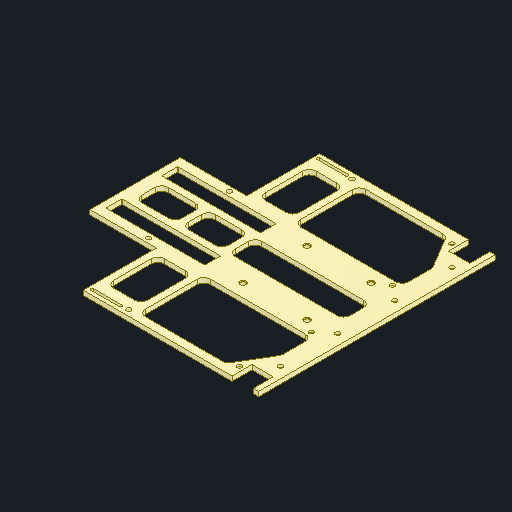
# Autodesk Inventor part: base
Saved by Autodesk Inventor 2023 (Build 270158000, 158)
## iProperties
Created: 2024-04-29
Part Number: base
Material: Nylon 6/6
Document SubType Name: Modeling
Designer: szymo
Density: 1.13 g/cm^3
Appearance: Nylon 6
Mass: 47.3407 g
Surface Area: 329.728 cm^2
Volume: 41.8944 cm^3
Author: szymo
Autodesk Inventor part; units mm, degrees
ref_plane "YZ Plane" through (0, 0, 0) normal (1, 0, 0) x (0, 1, 0)
ref_plane "XZ Plane" through (0, 0, 0) normal (0, 1, 0) x (-1, 0, 0)
ref_plane "XY Plane" through (0, 0, 0) normal (0, 0, 1) x (1, 0, 0)
sketch "Sketch1" plane through (0, 0, 0) normal (0, 1, 0) x (-1, 0, 0)
  line L0 (99, 89) -> (-99, 89)
  line L1 (-99, 89) -> (-99, -89)
  line L2 (-99, -89) -> (99, -89)
  line L3 (99, -89) -> (99, 89)
  line L4 (99, 89) -> (-99, -89) construction
  line L5 (-99, 89) -> (99, -89) construction
  line L6 (-99, 89) -> (-85, 89)
  line L7 (-85, 89) -> (-85, -89)
  line L8 (-85, -89) -> (-99, -89)
  line L9 (-99, -89) -> (-99, 89)
  line L10 (99, 89) -> (97, 89)
  line L11 (97, 89) -> (97, -89)
  line L12 (97, -89) -> (99, -89)
  line L13 (99, -89) -> (99, 89)
  line L14 (97, 33) -> (97, 35)
  line L15 (97, -33) -> (97, -35)
  line L16 (97, 32.8) -> (97, 35)
  line L17 (97, -32.8) -> (97, -35)
  line L18 (97, 89) -> (47, 89)
  line L19 (47, 89) -> (47, 34)
  line L20 (47, 34) -> (97, 34)
  line L21 (97, 34) -> (97, 89)
  line L22 (97, -89) -> (47, -89)
  line L23 (47, -89) -> (47, -34)
  line L24 (47, -34) -> (97, -34)
  line L25 (97, -34) -> (97, -89)
  line L26 (66.5, 33) -> (77.5, 33) projected
  line L27 (77.5, -33) -> (66.5, -33) projected
  line L28 (-81, 74) -> (-81, 89) projected
  line L29 (-81, 31) -> (-81, 55) projected
  line L30 (-81, -12) -> (-81, 12) projected
  line L31 (-81, -55) -> (-81, -31) projected
  line L32 (-81, -89) -> (-81, -74) projected
  arc A0 (-81, 74) -> (-79, 72) centre (-79, 74) ccw projected
  line L33 (-70, 72) -> (-79, 72) projected
  line L34 (-70, 57) -> (-70, 72) projected
  line L35 (-79, 57) -> (-70, 57) projected
  arc A1 (-79, 57) -> (-81, 55) centre (-79, 55) ccw projected
  arc A2 (-81, 31) -> (-79, 29) centre (-79, 31) ccw projected
  line L36 (-70, 29) -> (-79, 29) projected
  line L37 (-70, 14) -> (-70, 29) projected
  line L38 (-79, 14) -> (-70, 14) projected
  arc A3 (-79, 14) -> (-81, 12) centre (-79, 12) ccw projected
  arc A4 (-81, -12) -> (-79, -14) centre (-79, -12) ccw projected
  line L39 (-70, -14) -> (-79, -14) projected
  line L40 (-70, -29) -> (-70, -14) projected
  line L41 (-79, -29) -> (-70, -29) projected
  arc A5 (-79, -29) -> (-81, -31) centre (-79, -31) ccw projected
  arc A6 (-81, -55) -> (-79, -57) centre (-79, -55) ccw projected
  line L42 (-70, -57) -> (-79, -57) projected
  line L43 (-70, -72) -> (-70, -57) projected
  line L44 (-79, -72) -> (-70, -72) projected
  arc A7 (-79, -72) -> (-81, -74) centre (-79, -74) ccw projected
  circle A8 centre (-77, -64.5) radius 1.2295 projected
  circle A9 centre (-77, -21.5) radius 1.2295 projected
  circle A10 centre (-77, 21.5) radius 1.2295 projected
  circle A11 centre (-77, 64.5) radius 1.2295 projected
  line L45 (-65, 89) -> (-79, 89)
  line L46 (-79, 89) -> (-79, 75)
  line L47 (-79, 75) -> (-65, 75)
  line L48 (-65, 75) -> (-65, 89)
  line L49 (-65, 89) -> (-81, 89)
  line L50 (-81, 89) -> (-81, 74)
  line L51 (-81, 74) -> (-65, 74)
  line L52 (-65, 74) -> (-65, 89)
  line L53 (-99, 0) -> (97, 0)
  line L54 (0, 0) -> (-99, 0) construction
  line L55 (-65, -89) -> (-79, -89)
  line L56 (-79, -89) -> (-79, -75)
  line L57 (-79, -75) -> (-65, -75)
  line L58 (-65, -75) -> (-65, -89)
  line L59 (-65, -89) -> (-81, -89)
  line L60 (-81, -89) -> (-81, -74)
  line L61 (-81, -74) -> (-65, -74)
  line L62 (-65, -74) -> (-65, -89)
  point P0 (47, 89)
  point P1 (47, -89)
  point P2 (97, 34)
  point P3 (-81, -89)
  point P4 (-79, -74)
  dimension "d0" = 198
  dimension "d1" = 178
  dimension "d2" = 14
  dimension "d3" = 2
  dimension "d16" = 50
  dimension "d17" = 55
  dimension "d18" = 50
  dimension "d19" = 55
  dimension "d20" = 1
  dimension "d21" = 1
  dimension "d22" = 14
  dimension "d23" = 14
  dimension "d24" = 2
  dimension "d25" = 1
  dimension "d26" = 2
  constraints: 88 end point, 14 parallel, 10 symmetric about line, 8 perpendicular, 8 point on line, 7 horizontal, 4 midpoint, 2 collinear
  measures "d0" distance of L2.end L1.end
  measures "d1" distance of L1.end L0.end
  measures "d2" distance of L7.end L8.end
  measures "d3" distance of L12.end L11.end
  measures "d16" distance of L20.end L19.end
  measures "d17" distance of L19.end L18.end
  measures "d18" distance of L23.end L24.end
  measures "d19" distance of L22.end L23.end
  measures "d20" distance between parallel lines of L20 L26
  measures "d21" distance between parallel lines of L27 L24
  measures "d22" distance of L47.end L46.end
  measures "d23" distance of L46.end L45.end
  measures "d24" distance between parallel lines of L28 L46
  measures "d25" distance between parallel lines of L47 L51
  measures "d26" distance between parallel lines of L33 L51
extrude "Extrusion1" add sketch "Sketch1" along normal blind 3.5 contours L19 L20 L11 L53 L30 A3 L38 L37 L36 A2 L29 A1 L35 L34 L33 A0 L51 L52 L48 L0 | L2 L58 L62 L61 A7 L44 L43 L42 A6 L31 A5 L41 L40 L39 A4 L30 L53 L11 L24 L23 | L28 A0 L33 L34 L35 A1 L29 A2 L36 L37 L38 A3 L30 L53 L7 L0 | L2 L7 L53 L30 A4 L39 L40 L41 A5 L31 A6 L42 L43 L44 A7 L32 | A8 | A9 | A10 | A11
sketch "Sketch3" plane through (0, 0, 0) normal (0, -1, 0) x (1, 0, 0)
  line L0 (65, -74) -> (65, -89)
  line L1 (81, -74) -> (65, -74)
  line L2 (81, -89) -> (81, -74)
  line L3 (85, -89) -> (81, -89)
  line L4 (85, 89) -> (85, -89)
  line L5 (81, 89) -> (85, 89)
  line L6 (81, 74) -> (81, 89)
  line L7 (65, 74) -> (81, 74)
  line L8 (65, 89) -> (65, 74)
  line L9 (-47, 89) -> (65, 89)
  line L10 (-47, 34) -> (-47, 89)
  line L11 (-97, 34) -> (-47, 34)
  line L12 (-97, -34) -> (-97, 34)
  line L13 (-47, -34) -> (-97, -34)
  line L14 (-47, -89) -> (-47, -34)
  line L15 (65, -89) -> (-47, -89)
  circle A0 centre (70, 80) radius 1.75
  line L16 (73, 82.75) -> (73, 77)
  line L17 (-47, 89) -> (81, 89)
  line L18 (-47, 89) -> (-47, 76.2)
  line L19 (-14.25, 87) -> (-14.25, 76.2)
  line L20 (58, 77) -> (58, 82.75)
  line L21 (73, 77) -> (58, 77)
  circle A1 centre (-17.4116, 84.6) radius 1.8
  circle A2 centre (61.5, 80) radius 1.8
  circle A3 centre (70, -83) radius 1.75
  line L22 (-21.635, -86.2) -> (-21.635, -84.2)
  line L23 (-45.325, -86.2) -> (-21.635, -86.2)
  line L24 (-45.325, -84.2) -> (-45.325, -86.2)
  line L25 (-21.635, -84.2) -> (-45.325, -84.2)
  line L26 (73, -77) -> (73, -89)
  line L27 (73, -77) -> (58, -77)
  line L28 (58, -77) -> (58, -83)
  line L29 (58, -83) -> (-14.925, -83)
  line L30 (-14.925, -83) -> (-14.925, -76.2)
  line L31 (-14.925, -76.2) -> (-47, -76.2)
  line L32 (-47, -89) -> (-47, -76.2)
  line L33 (-47, -89) -> (73, -89)
  circle A4 centre (-18.3706, -84.6) radius 1.8
  circle A5 centre (61.5, -80) radius 1.8
  line L34 (-16.25, -37.7) -> (-47, -37.7)
  line L35 (-16.25, -37.7) -> (-16.25, -34.2)
  line L36 (-47, -37.7) -> (-47, -34.2)
  circle A6 centre (66.25, -30.5) radius 1.8
  circle A7 centre (-56.325, -30.5) radius 1.8
  line L37 (69.5, -34) -> (69.5, -27)
  line L38 (69.5, -27) -> (-97, -27)
  line L39 (-97, -27) -> (-97, -34)
  line L40 (-97, -34) -> (-94, -34)
  line L41 (-94, -34) -> (41.0514, -34)
  line L42 (41.0514, -34) -> (41.0514, -45)
  line L43 (41.0514, -45) -> (45.7494, -45)
  line L44 (45.7494, -45) -> (45.7494, -34.8203)
  line L45 (45.7494, -45) -> (59.075, -45)
  line L46 (59.075, -34) -> (59.075, -45)
  line L47 (59.075, -34) -> (69.5, -34)
  line L48 (-16.65, -10) -> (-16.65, -27)
  line L49 (-16.65, -10) -> (-97, -10)
  line L50 (-97, -15) -> (-97, -10)
  line L51 (-97, -15) -> (-18.65, -15)
  line L52 (-17.65, -16) -> (-17.65, -27)
  line L53 (-16.65, -27) -> (-17.65, -27)
  line L54 (-16.65, 10) -> (-16.65, 27)
  line L55 (-16.65, 27) -> (-17.65, 27)
  line L56 (-17.65, 16) -> (-17.65, 27)
  line L57 (-97, 15) -> (-18.65, 15)
  line L58 (-97, 15) -> (-97, 10)
  line L59 (-16.65, 10) -> (-97, 10)
  line L60 (-47, 37.7) -> (-47, 34.2)
  line L61 (-16.25, 37.7) -> (-16.25, 34.2)
  circle A8 centre (66.25, 30.5) radius 1.8
  circle A9 centre (-56.325, 30.5) radius 1.8
  line L62 (69.5, 34) -> (69.5, 27)
  line L63 (-97, 34) -> (-94, 34)
  line L64 (59.075, 37) -> (59.075, 45)
  line L65 (45.7494, 45) -> (59.075, 45)
  line L66 (45.7494, 45) -> (45.7494, 34.8203)
  line L67 (41.0514, 45) -> (45.7494, 45)
  line L68 (41.0514, 36) -> (41.0514, 45)
  line L69 (-97, 27) -> (-97, 34)
  line L70 (69.5, 27) -> (-97, 27)
  circle A10 centre (77, 21.5) radius 1.2295
  circle A11 centre (77, -64.5) radius 1.2295
  circle A12 centre (77, -21.5) radius 1.2295
  circle A13 centre (77, 64.5) radius 1.2295
  line L71 (70, -72) -> (79, -72)
  arc A14 (81, -74) -> (79, -72) centre (79, -74) ccw
  line L72 (81, -74) -> (81, -89)
  line L73 (81, -89) -> (85, -89)
  line L74 (85, -89) -> (85, 89)
  line L75 (81, 89) -> (85, 89)
  line L76 (81, 89) -> (81, 74)
  arc A15 (79, 72) -> (81, 74) centre (79, 74) ccw
  line L77 (79, 72) -> (70, 72)
  line L78 (70, 57) -> (70, 72)
  line L79 (70, 57) -> (79, 57)
  arc A16 (81, 55) -> (79, 57) centre (79, 55) ccw
  line L80 (81, 55) -> (81, 31)
  arc A17 (79, 29) -> (81, 31) centre (79, 31) ccw
  line L81 (79, 29) -> (70, 29)
  line L82 (70, 14) -> (70, 29)
  line L83 (70, 14) -> (79, 14)
  arc A18 (81, 12) -> (79, 14) centre (79, 12) ccw
  line L84 (81, 12) -> (81, -12)
  arc A19 (79, -14) -> (81, -12) centre (79, -12) ccw
  line L85 (79, -14) -> (70, -14)
  line L86 (70, -29) -> (70, -14)
  line L87 (70, -29) -> (79, -29)
  arc A20 (81, -31) -> (79, -29) centre (79, -31) ccw
  line L88 (81, -31) -> (81, -55)
  arc A21 (79, -57) -> (81, -55) centre (79, -55) ccw
  line L89 (79, -57) -> (70, -57)
  line L90 (70, -72) -> (70, -57)
  line L91 (85, 89) -> (70, 89)
  line L92 (70, 89) -> (70, -89)
  line L93 (65, -89) -> (85, -89)
  line L94 (85, -89) -> (85, 89)
  line L95 (85, 34) -> (-97, 34)
  line L96 (-97, 34) -> (-97, 10)
  line L97 (-97, 10) -> (85, 10)
  line L98 (85, 10) -> (85, 34)
  line L99 (-97, -10) -> (85, -10)
  line L100 (85, -10) -> (85, -34)
  line L101 (85, -34) -> (-97, -34)
  line L102 (-97, -34) -> (-97, -10)
  line L103 (-47, 34) -> (-47, 34.2)
  line L104 (-47, 34.2) -> (-97, 34)
  line L105 (-97, -34) -> (-47, -34.2)
  line L106 (-47, -34.2) -> (-47, -34)
  line L107 (70, 89) -> (58, 89)
  line L108 (58, 89) -> (58, 77)
  line L109 (58, 77) -> (70, 77)
  line L110 (70, 77) -> (70, 89)
  line L111 (58, 89) -> (-14.925, 89)
  line L112 (-14.925, 89) -> (-14.925, 83)
  line L113 (-14.925, 83) -> (58, 83)
  line L114 (58, 83) -> (58, 89)
  line L115 (-14.925, 89) -> (-47, 89)
  line L116 (-47, 89) -> (-47, 76.2)
  line L117 (-47, 76.2) -> (-14.925, 76.2)
  line L118 (-14.925, 76.2) -> (-14.925, 89)
  line L119 (65, -77) -> (58, -77)
  line L120 (58, -77) -> (58, -89)
  line L121 (58, -89) -> (70, -89)
  line L122 (70, -89) -> (70, -77)
  line L123 (58, -89) -> (-14.925, -89)
  line L124 (-14.925, -89) -> (-14.925, -83)
  line L125 (-14.925, -83) -> (58, -83)
  line L126 (58, -83) -> (58, -89)
  line L127 (-14.925, -89) -> (-47, -89)
  line L128 (-47, -89) -> (-47, -76.2)
  line L129 (-47, -76.2) -> (-14.925, -76.2)
  line L130 (-14.925, -76.2) -> (-14.925, -89)
  line L131 (-47, -76.2) -> (-42, -76.2)
  line L132 (-42, -76.2) -> (-42, -34)
  line L133 (-42, -34) -> (-47, -34)
  line L134 (-47, -34) -> (-47, -76.2)
  line L135 (-47, 76.2) -> (-42, 76.2)
  line L136 (-42, 76.2) -> (-42, 34)
  line L137 (-42, 34) -> (-47, 34)
  line L138 (-47, 34) -> (-47, 76.2)
  line L139 (-16.25, 34.2) -> (-11.25, 34.2)
  line L140 (-11.25, 34.2) -> (-11.25, 83)
  line L141 (-11.25, 83) -> (-16.25, 83)
  line L142 (-16.25, 83) -> (-16.25, 34.2)
  line L143 (-16.25, -34.2) -> (-11.25, -34.2)
  line L144 (-11.25, -34.2) -> (-11.25, -83)
  line L145 (-11.25, -83) -> (-16.25, -83)
  line L146 (-16.25, -83) -> (-16.25, -34.2)
  line L147 (-16.65, 10) -> (-21.65, 10)
  line L148 (-21.65, 10) -> (-21.65, -10)
  line L149 (-21.65, -10) -> (-16.65, -10)
  line L150 (-16.65, -10) -> (-16.65, 10)
  line L151 (-97, 10) -> (-87, 10)
  line L152 (-87, 10) -> (-87, -10)
  line L153 (-87, -10) -> (-97, -10)
  line L154 (-97, -10) -> (-97, 10)
  line L155 (-51.825, 10) -> (-56.825, 10)
  line L156 (-56.825, 10) -> (-56.825, -10)
  line L157 (-56.825, -10) -> (-51.825, -10)
  line L158 (-51.825, -10) -> (-51.825, 10)
  line L159 (-16.25, 34.2) -> (-16.25, 34)
  line L160 (-11.25, 34.2) -> (-11.25, 34)
  line L161 (-11.25, -34.2) -> (-11.25, -34)
  line L162 (-16.25, -34.2) -> (-16.25, -34)
  line L163 (70, 57) -> (54.4, 83)
  line L164 (70, -57) -> (54.4, -83)
  line L165 (-34.0117, 16) -> (-34.0117, 26)
  line L166 (-34.0117, 26) -> (-32.704, 26)
  line L167 (-32.704, 26) -> (-32.704, 16)
  line L168 (-32.704, 16) -> (-34.0117, 16)
  line L169 (-35.6343, 26) -> (-35.6343, 16)
  line L170 (-35.6343, 16) -> (-50.4468, 16)
  line L171 (-50.4468, 16) -> (-50.4468, 26)
  line L172 (-50.4468, 26) -> (-35.6343, 26)
  line L173 (-66.4245, 19) -> (-72.4408, 19)
  line L174 (-72.4408, 19) -> (-72.4408, 23)
  line L175 (-72.4408, 23) -> (-66.4245, 23)
  line L176 (-66.4245, 23) -> (-66.4245, 19)
  line L177 (-82.583, 26) -> (-82.583, 23)
  line L178 (-82.583, 23) -> (-80.9671, 23)
  line L179 (-80.9671, 23) -> (-80.9671, 19)
  line L180 (-80.9671, 19) -> (-82.583, 19)
  line L181 (-82.583, 19) -> (-82.583, 16)
  line L182 (-82.583, 16) -> (-86.007, 16)
  spline S0 degree 3 poles (-86.007, 16) (-86.007, 17.6667) (-86.007, 19.3333) (-86.007, 22.6667) (-86.007, 24.3333) (-86.007, 26) knots -1 -1 -1 -1 -0.5 -0.5 0 0 0 0
  line L183 (-86.007, 26) -> (-82.583, 26)
  line L184 (-61.417, 23) -> (-61.417, 26)
  line L185 (-61.417, 26) -> (-57.3554, 26)
  spline S1 degree 3 poles (-57.3554, 26) (-57.3554, 24.3333) (-57.3554, 22.6667) (-57.3554, 19.3333) (-57.3554, 17.6667) (-57.3554, 16) knots -1 -1 -1 -1 -0.5 -0.5 0 0 0 0
  line L186 (-57.3554, 16) -> (-61.417, 16)
  line L187 (-61.417, 16) -> (-61.417, 19)
  line L188 (-61.417, 19) -> (-62.6269, 19)
  line L189 (-62.6269, 19) -> (-62.6269, 23)
  line L190 (-62.6269, 23) -> (-61.417, 23)
  line L191 (-57.2691, 26) -> (-57.2691, 16)
  line L192 (-86.7309, 16) -> (-86.7309, 26)
  line L193 (-49.6101, -16) -> (-49.6101, -26)
  line L194 (-49.6101, -26) -> (-51.9631, -26)
  line L195 (-51.9631, -26) -> (-51.9631, -16)
  line L196 (-51.9631, -16) -> (-49.6101, -16)
  line L197 (-33.7735, -16) -> (-33.7735, -26)
  line L198 (-33.7735, -26) -> (-49.1385, -26)
  line L199 (-49.1385, -26) -> (-49.1385, -16)
  line L200 (-49.1385, -16) -> (-33.7735, -16)
  line L201 (-61.417, -26) -> (-61.417, -23)
  line L202 (-61.417, -23) -> (-69.2128, -23)
  line L203 (-69.2128, -23) -> (-69.2128, -19)
  line L204 (-69.2128, -19) -> (-61.417, -19)
  line L205 (-61.417, -19) -> (-61.417, -16)
  line L206 (-61.417, -16) -> (-57.0283, -16)
  spline S2 degree 3 poles (-57.0283, -16) (-57.0283, -17.6667) (-57.0283, -19.3333) (-57.0283, -22.6667) (-57.0283, -24.3333) (-57.0283, -26) knots -1 -1 -1 -1 -0.5 -0.5 0 0 0 0
  line L207 (-57.0283, -26) -> (-61.417, -26)
  line L208 (-82.583, -23) -> (-82.583, -26)
  line L209 (-82.583, -26) -> (-85.6557, -26)
  spline S3 degree 3 poles (-85.6557, -26) (-85.6557, -24.3333) (-85.6557, -22.6667) (-85.6557, -19.3333) (-85.6557, -17.6667) (-85.6557, -16) knots -1 -1 -1 -1 -0.5 -0.5 0 0 0 0
  line L210 (-85.6557, -16) -> (-82.583, -16)
  line L211 (-82.583, -16) -> (-82.583, -19)
  line L212 (-82.583, -19) -> (-78.6331, -19)
  line L213 (-78.6331, -19) -> (-78.6331, -23)
  line L214 (-78.6331, -23) -> (-82.583, -23)
  line L215 (-57.2691, -16) -> (-57.2691, -26)
  line L216 (-86.7309, -26) -> (-86.7309, -16)
  line L217 (-27.704, 27) -> (-27.704, 15)
  line L218 (-92, 15) -> (-92, 27)
  line L219 (-92, -15) -> (-92, -27)
  line L220 (-28.7735, -15) -> (-28.7735, -27)
  line L221 (62.075, 34) -> (69.5, 34)
  arc A22 (59.075, 37) -> (62.075, 34) centre (62.075, 37) ccw
  arc A23 (39.0514, 34) -> (41.0514, 36) centre (39.0514, 36) ccw
  line L222 (-94, 34) -> (39.0514, 34)
  line L223 (81, 87) -> (77.25, 87)
  line L224 (81, 89) -> (81, 87)
  line L225 (53.75, 87) -> (-14.25, 87)
  arc A24 (58, 82.75) -> (53.75, 87) centre (53.75, 82.75) ccw
  arc A25 (77.25, 87) -> (73, 82.75) centre (77.25, 82.75) ccw
  line L226 (-14.25, 76.2) -> (-47, 76.2)
  line L227 (-97, -34) -> (-97, 34)
  line L228 (-97, 0) -> (85, 0) construction
  line L229 (-17.65, -16) -> (-17.65, -15)
  line L230 (-17.65, -15) -> (-18.65, -15)
  line L231 (-17.65, 16) -> (-17.65, 15)
  line L232 (-17.65, 15) -> (-18.65, 15)
  line L233 (-21.635, 86.2) -> (-21.635, 84.2)
  line L234 (-45.325, 86.2) -> (-21.635, 86.2)
  line L235 (-45.325, 84.2) -> (-45.325, 86.2)
  line L236 (-21.635, 84.2) -> (-45.325, 84.2)
  line L237 (-16.25, -34.2) -> (-47, -34.2)
  line L238 (-16.25, 34.2) -> (-47, 34.2)
  line L239 (-16.5, 38) -> (-47, 38)
  line L240 (-47, 38) -> (-47, 34.2)
  line L241 (-16.5, 38) -> (-16.5, 34.2)
  line L242 (-16.5, -38) -> (-47, -38)
  line L243 (-16.5, -38) -> (-16.5, -34.2)
  line L244 (-47, -38) -> (-47, -34.2)
  line L245 (70, -27) -> (69.5, -27)
  line L246 (70, 27) -> (69.5, 27)
  line L247 (-16.5, 38) -> (-16.25, 38)
  line L248 (-16.5, -38) -> (-16.25, -38)
  line L249 (-16.5, -34.2) -> (-47, -34.2)
  line L250 (-16.5, 34.2) -> (-47, 34.2)
  point P0 (0, 0)
  point P1 (-16.25, -76.2)
  point P2 (-42, -37.7)
  point P3 (-87, -10)
  point P4 (70, -10)
  point P5 (70, 10)
  point P6 (70, -34)
  point P7 (70, 34)
  point P8 (41.0514, 34)
  point P9 (59.075, 34)
  point P10 (39.0514, 34)
  point P11 (70, 77)
  point P12 (-16.25, 35.2)
  point P13 (-16.25, 76.2)
  point P14 (-42, 38)
  point P15 (-42, -38)
extrude "Extrusion2" cut sketch "Sketch3" against normal up to next contours L164 L29 L144 L161 L41 L42 L43 L45 L46 L47 L101 L92 | L46 L45 L43 L42 L101 | L132 L242 L248 L146 L31 | L99 L150 L97 L92 | L38 L220 L51 L230 L229 L52 | L38 L219 L51 L220 | L49 L158 L59 L148 | L95 A22 L64 L65 L67 L68 A23 L160 L140 L113 L163 L92 | L49 L152 L59 L156 | L56 L231 L232 L57 L217 L70 | L217 L57 L218 L70 | L95 A23 L68 L67 L65 L64 A22 | L117 L142 L247 L239 L136 | L23 L24 L25 L22 | L165 L166 L167 L168 | L169 L170 L171 L172 | L173 L174 L175 L176 | L177 L178 L179 L180 L181 L182 S0 L183 | L184 L185 S1 L186 L187 L188 L189 L190 | L193 L194 L195 L196 | L197 L198 L199 L200 | L201 L202 L203 L204 L205 L206 L215 L207 | L215 L206 S2 L207 | L208 L209 S3 L210 L211 L212 L213 L214 | L233 L236 L235 L234
sketch "Sketch4" plane through (0, 0, 0) normal (0, -1, 0) x (1, 0, 0)
  circle A0 centre (-56.325, -30.5) radius 3 projected
  circle A1 centre (66.25, -30.5) radius 1.8 projected
  circle A2 centre (61.5, -80) radius 1.8 projected
  circle A3 centre (61.5, 80) radius 1.8 projected
  circle A4 centre (-17.2102, 84.6) radius 1.8 projected
  circle A5 centre (-18.3706, -84.6) radius 1.8 projected
  circle A6 centre (8.4, 24.1) radius 1.6 projected
  circle A7 centre (8.4, -24.1) radius 1.6 projected
  circle A8 centre (56.6, -24.1) radius 1.6 projected
  circle A9 centre (56.6, 24.1) radius 1.6 projected
  point P0 (0, 0)
  point P1 (-56.325, 30.5)
  point P2 (66.25, 30.5)
  constraints: 10 coincident
hole "Hole1" at (-56.325, 0, -30.5) at (-56.325, 0, 30.5) at (-17.2102, 0, 84.6) at (-18.3706, 0, -84.6) at (61.5, 0, 80) at (66.25, 0, 30.5) at (66.25, 0, -30.5) at (61.5, 0, -80) direction (0, 1, 0) diameter 3.6 end through all counterbore diameter 11 counterbore depth 0 clearance for "Hex Head Cap Screw ISO 24014 (Spotface)" size "M3" standard "ISO"
sketch "Sketch5" plane through (0, 0, 0) normal (0, -1, 0) x (1, 0, 0)
  circle A0 centre (77, 21.5) radius 1.2295 projected
  circle A1 centre (77, -64.5) radius 1.2295 projected
  circle A2 centre (77, -21.5) radius 1.2295 projected
  circle A3 centre (77, 64.5) radius 1.2295 projected
  line L0 (79, -72) -> (70, -72) projected
  line L1 (70, -72) -> (70, -57) projected
  line L2 (70, -57) -> (79, -57) projected
  arc A4 (79, -57) -> (81, -55) centre (79, -55) ccw projected
  line L3 (81, -55) -> (81, -31) projected
  arc A5 (81, -31) -> (79, -29) centre (79, -31) ccw projected
  line L4 (79, -29) -> (70, -29) projected
  line L5 (70, -29) -> (70, -14) projected
  line L6 (70, -14) -> (79, -14) projected
  arc A6 (79, -14) -> (81, -12) centre (79, -12) ccw projected
  line L7 (81, -12) -> (81, 12) projected
  arc A7 (81, 12) -> (79, 14) centre (79, 12) ccw projected
  line L8 (79, 14) -> (70, 14) projected
  line L9 (70, 14) -> (70, 29) projected
  line L10 (70, 29) -> (79, 29) projected
  arc A8 (79, 29) -> (81, 31) centre (79, 31) ccw projected
  line L11 (81, 31) -> (81, 55) projected
  arc A9 (81, 55) -> (79, 57) centre (79, 55) ccw projected
  line L12 (79, 57) -> (70, 57) projected
  line L13 (70, 57) -> (70, 72) projected
  line L14 (70, 72) -> (79, 72) projected
  arc A10 (79, 72) -> (81, 74) centre (79, 74) ccw projected
  line L15 (81, 74) -> (81, 89) projected
  line L16 (85, 89) -> (81, 89) projected
  line L17 (85, -89) -> (85, 89) projected
  line L18 (85, -89) -> (81, -89) projected
  line L19 (81, -89) -> (81, -74) projected
  arc A11 (81, -74) -> (79, -72) centre (79, -74) ccw projected
  point P0 (0, 0)
  constraints: 4 coincident
hole "Hole2" at (77, 0, -64.5) at (77, 0, -21.5) at (77, 0, 21.5) at (77, 0, 64.5) direction (0, 1, 0) diameter 3.6 end through all countersink diameter 6.7 countersink angle 90
sketch "Sketch6" plane through (0, 0, 0) normal (0, -1, 0) x (1, 0, 0)
  circle A0 centre (-56.325, -30.5) radius 1.8 projected
  circle A1 centre (-56.325, 30.5) radius 1.8 projected
  circle A2 centre (-17.2102, 84.6) radius 1.8 projected
  circle A3 centre (-18.3706, -84.6) radius 1.8 projected
  circle A4 centre (8.4, -24.1) radius 1.8
  circle A5 centre (8.4, 24.1) radius 1.8
  circle A6 centre (56.6, 24.1) radius 1.8
  circle A7 centre (66.25, 30.5) radius 1.8 projected
  circle A8 centre (61.5, 80) radius 1.8 projected
  circle A9 centre (56.6, -24.1) radius 1.8
  circle A10 centre (66.25, -30.5) radius 1.8 projected
  circle A11 centre (61.5, -80) radius 1.8 projected
  line L0 (-53.0341, -30.5) -> (-54.6796, -33.35)
  line L1 (-54.6796, -33.35) -> (-57.9704, -33.35)
  line L2 (-57.9704, -33.35) -> (-59.6159, -30.5)
  line L3 (-59.6159, -30.5) -> (-57.9704, -27.65)
  line L4 (-57.9704, -27.65) -> (-54.6796, -27.65)
  line L5 (-54.6796, -27.65) -> (-53.0341, -30.5)
  line L6 (-53.0341, 30.5) -> (-54.6796, 27.65)
  line L7 (-54.6796, 27.65) -> (-57.9704, 27.65)
  line L8 (-57.9704, 27.65) -> (-59.6159, 30.5)
  line L9 (-59.6159, 30.5) -> (-57.9704, 33.35)
  line L10 (-57.9704, 33.35) -> (-54.6796, 33.35)
  line L11 (-54.6796, 33.35) -> (-53.0341, 30.5)
  line L12 (-14.3716, 82.935) -> (-17.2328, 81.3092)
  line L13 (-17.2328, 81.3092) -> (-20.0714, 82.9741)
  line L14 (-20.0714, 82.9741) -> (-20.0488, 86.265)
  line L15 (-20.0488, 86.265) -> (-17.1876, 87.8908)
  line L16 (-17.1876, 87.8908) -> (-14.349, 86.2259)
  line L17 (-14.349, 86.2259) -> (-14.3716, 82.935)
  line L18 (-15.5328, -86.2664) -> (-18.3949, -87.8908)
  line L19 (-18.3949, -87.8908) -> (-21.2326, -86.2244)
  line L20 (-21.2326, -86.2244) -> (-21.2084, -82.9336)
  line L21 (-21.2084, -82.9336) -> (-18.3463, -81.3092)
  line L22 (-18.3463, -81.3092) -> (-15.5085, -82.9756)
  line L23 (-15.5085, -82.9756) -> (-15.5328, -86.2664)
  point P0 (0, 0)
  point P1 (-15.5207, -84.621)
  dimension "d61" = 5.7
  dimension "d62" = 5.7
  dimension "d63" = 5.7
  dimension "d64" = 5.7
  constraints: 48 end point, 4 centre point, 4 coincident, 1 midpoint, 1 point on line, 52 other
  measures "d61" distance between parallel lines of L22 L19
  measures "d62" distance between parallel lines of L4 L1
  measures "d63" distance between parallel lines of L10 L7
  measures "d64" distance between parallel lines of L16 L13
extrude "Extrusion3" cut sketch "Sketch6" against normal blind 0.5 contours L0 L1 L2 L3 L4 L5 | L6 L7 L8 L9 L10 L11 | L12 L13 L14 L15 L16 L17 | L18 L19 L20 L21 L22 L23
sketch "Sketch7" plane through (0, 0, 0) normal (0, -1, 0) x (1, 0, 0)
  circle A0 centre (66.25, 30.5) radius 1.8 projected
  circle A1 centre (61.5, 80) radius 1.8 projected
  circle A2 centre (66.25, -30.5) radius 1.8 projected
  circle A3 centre (61.5, -80) radius 1.8 projected
  line L0 (58.65, -78.3546) -> (61.5, -76.7091)
  line L1 (61.5, -76.7091) -> (64.35, -78.3546)
  line L2 (64.35, -78.3546) -> (64.35, -81.6454)
  line L3 (64.35, -81.6454) -> (61.5, -83.2909)
  line L4 (61.5, -83.2909) -> (58.65, -81.6454)
  line L5 (58.65, -81.6454) -> (58.65, -78.3546)
  line L6 (58.6536, 81.6517) -> (61.5072, 83.2909)
  line L7 (61.5072, 83.2909) -> (64.3536, 81.6392)
  line L8 (64.3536, 81.6392) -> (64.3464, 78.3483)
  line L9 (64.3464, 78.3483) -> (61.4928, 76.7091)
  line L10 (61.4928, 76.7091) -> (58.6464, 78.3608)
  line L11 (58.6464, 78.3608) -> (58.6536, 81.6517)
  line L12 (64.6046, 27.65) -> (62.9591, 30.5)
  line L13 (62.9591, 30.5) -> (64.6046, 33.35)
  line L14 (64.6046, 33.35) -> (67.8954, 33.35)
  line L15 (67.8954, 33.35) -> (69.5409, 30.5)
  line L16 (69.5409, 30.5) -> (67.8954, 27.65)
  line L17 (67.8954, 27.65) -> (64.6046, 27.65)
  line L18 (67.8954, -27.65) -> (69.5409, -30.5)
  line L19 (69.5409, -30.5) -> (67.8954, -33.35)
  line L20 (67.8954, -33.35) -> (64.6046, -33.35)
  line L21 (64.6046, -33.35) -> (62.9591, -30.5)
  line L22 (62.9591, -30.5) -> (64.6046, -27.65)
  line L23 (64.6046, -27.65) -> (67.8954, -27.65)
  point P0 (56.6, 24.1)
  point P1 (58.65, 80.0062)
  dimension "d71" = 5.7
  dimension "d72" = 5.7
  dimension "d73" = 5.7
  dimension "d74" = 5.7
  constraints: 48 end point, 4 coincident, 1 midpoint, 1 point on line, 52 other
  measures "d71" distance between parallel lines of L7 L10
  measures "d72" distance between parallel lines of L14 L17
  measures "d73" distance between parallel lines of L23 L20
  measures "d74" distance between parallel lines of L1 L4
extrude "Extrusion4" cut sketch "Sketch7" against normal blind 2
fillet "Fillet1" radius 5 30 edges at (-87, 1.75, -10) (-87, 1.75, 10) (-56.825, 1.75, 10) (-56.825, 1.75, -10) (-51.825, 1.75, -10) (-51.825, 1.75, 10) (-21.65, 1.75, 10) (-21.65, 1.75, -10) (-16.65, 1.75, -10) (-16.65, 1.75, 10) (70, 1.75, 10) (70, 1.75, -10) (70, 1.75, 34) (70, 1.75, 57) (-42, 1.75, -76.2) (-16.25, 1.75, -76.2) (-11.25, 1.75, -34) (70, 1.75, -34) (70, 1.75, -57) (54.4, 1.75, -83) (-11.25, 1.75, -83) (54.4, 1.75, 83) (-11.25, 1.75, 83) (-11.25, 1.75, 34) (-42, 1.75, 76.2) (-16.25, 1.75, 76.2) (-42, 1.75, -38) (-16.25, 1.75, -38) (-16.25, 1.75, 38) (-42, 1.75, 38)
fillet "Fillet2" radius 0.4 8 edges at (-92, 1.75, -27) (-92, 1.75, -15) (-92, 1.75, 15) (-92, 1.75, 27) (-17.65, 1.75, -27) (-17.65, 1.75, 27) (-17.65, 1.75, -15) (-17.65, 1.75, 15)
fillet "Fillet3" radius 1 8 edges at (-45.325, 1.75, -86.2) (-45.325, 1.75, -84.2) (-21.635, 1.75, -86.2) (-21.635, 1.75, -84.2) (-45.325, 1.75, 84.2) (-45.325, 1.75, 86.2) (-21.635, 1.75, 84.2) (-21.635, 1.75, 86.2)
sketch "Sketch8" plane through (0, 3.5, 0) normal (0, 1, 0) x (1, 0, 0)
  circle A0 centre (8.4, -24.1) radius 1.6 projected
  circle A1 centre (8.4, 24.1) radius 1.6 projected
  circle A2 centre (56.6, 24.1) radius 1.6 projected
  circle A3 centre (56.6, -24.1) radius 1.6 projected
  point P0 (0, 0)
hole "Hole3" at (8.4, 3.5, 24.1) at (8.4, 3.5, -24.1) at (56.6, 3.5, -24.1) at (56.6, 3.5, 24.1) direction (0, -1, 0) diameter 4 depth 3.75 counterbore diameter 4.6 counterbore depth 0.75
equation "\"d34\" = d35"
equation "\"d35\" = 30.175"
body "Solid1"
